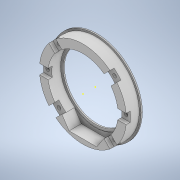
# Autodesk Inventor part: LCDmount
Saved by Autodesk Inventor 2022 (Build 260153000, 153)
## iProperties
Created: 2023-10-26
Part Number: LCDmount
Material: Generisch
Document SubType Name: Modeling
Designer: Marc Panse
Density: 1 g/cm^3
Appearance: Vorgabe
Author: Marc Panse
## iProperties of the stored document LCDmount_3D-Druck.ipt
Created: 2023-10-26
Part Number: LCDmount_3D-Druck
Material: Generisch
Document SubType Name: Modeling
Designer: Marc Panse
Density: 1 g/cm^3
Appearance: Vorgabe
Author: Marc Panse
Autodesk Inventor part; units mm, degrees
ref_plane "YZ Plane" through (0, 0, 0) normal (1, 0, 0) x (0, 1, 0)
ref_plane "XZ Plane" through (0, 0, 0) normal (0, 1, 0) x (-1, 0, 0)
ref_plane "XY Plane" through (0, 0, 0) normal (0, 0, 1) x (1, 0, 0)
sketch "Skizze1" plane through (0, 0, 0) normal (0, 0, 1) x (1, 0, 0)
  circle A0 centre (0, 0) radius 18
  circle A1 centre (0, 0) radius 25
  dimension "d0" = 36
  dimension "d1" = 50
  constraints: 2 centre point, 2 coincident
  measures "d0" diameter of A0
  measures "d1" diameter of A1
extrude "Extrusion1" add sketch "Skizze1" along normal blind 35
sketch "Skizze2" plane through (0, 0, 35) normal (0, 0, 1) x (1, 0, 0)
  circle A0 centre (0, 0) radius 19.3
  line L0 (0, -19.3) -> (0, -21.4)
  line L1 (0, -21.4) -> (-7.65, -21.4)
  line L2 (-7.65, -21.4) -> (7.65, -21.4)
  line L3 (7.65, -21.4) -> (7.65, -17.7191)
  line L4 (-7.65, -21.4) -> (-7.65, -17.7191)
  circle A1 centre (0, 0) radius 25 projected
  circle A2 centre (0, 0) radius 18 projected
  circle A3 centre (0, 0) radius 25 projected
  circle A4 centre (0, 0) radius 18 projected
  circle A5 centre (0, 0) radius 19.3
  dimension "d4" = 38.6
  dimension "d5" = 2.1
  dimension "d6" = 7.65
  dimension "d7" = 90
  dimension "d8" = 15.3
  constraints: 10 end point, 3 point on circle, 2 centre point, 2 coincident, 2 perpendicular, 1 concentric, 1 parallel, 1 point on line, 1 vertical
  measures "d4" diameter of A0
  measures "d5" distance of L0.start L0.end
  measures "d6" distance of L0.end L1.end
  measures "d7" angle of L0 L1
  measures "d8" distance of L1.end L2.end
extrude "Extrusion2" cut sketch "Skizze2" against normal blind 34 contours A0 | A0 L0 L1 L4 | L3 L2 L0 A0 | A2
fillet "Rundung1" radius 4 2 edges at (-7.65, -17.7191, 18) (7.65, -17.7191, 18)
sketch "Skizze3" plane through (0, 0, 35) normal (0, 0, 1) x (1, 0, 0)
  arc A0 (9.65, -16.7143) -> (7.65, -20.1784) centre (11.65, -20.1784) ccw projected
  line L0 (7.65, -20.1784) -> (7.65, -21.4) projected
  line L1 (7.65, -21.4) -> (-7.65, -21.4) projected
  line L2 (-7.65, -21.4) -> (-7.65, -20.1784) projected
  arc A1 (-7.65, -20.1784) -> (-9.65, -16.7143) centre (-11.65, -20.1784) ccw projected
  arc A2 (9.65, -16.7143) -> (-9.65, -16.7143) centre (0, 0) ccw projected
  circle A3 centre (0, 0) radius 25 projected
extrude "Extrusion3" cut sketch "Skizze3" against normal blind 25
sketch "Skizze4" plane through (0, 0, 10) normal (0, 0, 1) x (1, 0, 0)
  circle A0 centre (0, 0) radius 24
  circle A1 centre (0, 0) radius 25 projected
  arc A2 (9.65, -16.7143) -> (7.65, -20.1784) centre (11.65, -20.1784) ccw projected
  line L0 (7.65, -21.4) -> (7.65, -20.1784) projected
  line L1 (-7.65, -21.4) -> (7.65, -21.4) projected
  line L2 (-7.65, -20.1784) -> (-7.65, -21.4) projected
  arc A3 (-7.65, -20.1784) -> (-9.65, -16.7143) centre (-11.65, -20.1784) ccw projected
  arc A4 (9.65, -16.7143) -> (-9.65, -16.7143) centre (0, 0) ccw projected
  dimension "d14" = 48
  constraints: 1 centre point, 1 coincident
  measures "d14" diameter of A0
extrude "Extrusion4" cut sketch "Skizze4" against normal blind 9.25 contours A1
sketch "Skizze5" plane through (0, 0, 10) normal (0, 0, 1) x (1, 0, 0)
  circle A0 centre (0, 0) radius 24 projected
  arc A1 (9.65, -16.7143) -> (7.65, -20.1784) centre (11.65, -20.1784) ccw projected
  line L0 (7.65, -21.4) -> (7.65, -20.1784) projected
  line L1 (-7.65, -21.4) -> (7.65, -21.4) projected
  line L2 (-7.65, -20.1784) -> (-7.65, -21.4) projected
  arc A2 (-7.65, -20.1784) -> (-9.65, -16.7143) centre (-11.65, -20.1784) ccw projected
  arc A3 (9.65, -16.7143) -> (-9.65, -16.7143) centre (0, 0) ccw projected
extrude "Extrusion5" cut sketch "Skizze5" against normal blind 2.2
sketch "Skizze6" plane through (0, 0, 7.8) normal (0, 0, 1) x (1, 0, 0)
  line L0 (30, -2.706) -> (-30, -2.706)
  line L1 (-30, -2.706) -> (-30, 2.706)
  line L2 (-30, 2.706) -> (30, 2.706)
  line L3 (30, 2.706) -> (30, -2.706)
  line L4 (30, -2.706) -> (-30, 2.706) construction
  line L5 (-30, -2.706) -> (30, 2.706) construction
  point P0 (0, 0)
  dimension "d33" = 60
  constraints: 12 end point, 2 midpoint, 2 parallel, 1 horizontal, 1 perpendicular
  measures "d33" distance between parallel lines of L3 L1
extrude "Extrusion6" cut sketch "Skizze6" against normal blind 2.2
sketch "Skizze7" plane through (0, 0, 5.6) normal (0, 0, 1) x (1, 0, 0)
  line L0 (-22.5614, -2.035) -> (-22.5614, 2.035) projected
  line L1 (-22.5614, 0) -> (-19.3, 0)
  arc A0 (-19.1094, 2.706) -> (-19.1094, -2.706) centre (0, 0) ccw projected
  line L2 (-19.3, 0) -> (-24, 0)
  circle A1 centre (0, 0) radius 24 projected
  circle A2 centre (-21.65, 0) radius 0.9
  dimension "d34" = 1.8
  constraints: 4 end point, 2 horizontal, 2 midpoint, 1 centre point, 1 horizontal alignment, 1 point on circle, 1 other
  measures "d34" diameter of A2
extrude "Extrusion7" cut sketch "Skizze7" against normal blind 4 contours A2 L1 | L1 A2
mirror "Spiegeln1" about plane through (0, 0, 0) normal (1, 0, 0) of "Extrusion7"
sketch "Skizze8" plane through (0, 0, 7.8) normal (0, 0, 1) x (1, 0, 0)
  point P0 (0, 0)
pattern_circular "Runde Anordnung1" count 8 over 360 about axis through (0, 0, -10) along (0, 0, 1) of "Extrusion7", "Extrusion6"
sketch "Skizze9" plane through (0, -20.9307, 1.6) normal (0, 0, 1) x (1, 0, 0)
  line L0 (-0.8646, -0.4693) -> (0.8646, -0.4693) projected
  line L1 (-2.706, -0.4693) -> (-0.8646, -0.4693) projected
  line L2 (-2.706, 40.0401) -> (-2.706, 44.7777) projected
  line L3 (2.706, 44.7777) -> (2.706, 40.0401) projected
  arc A0 (2.706, 44.7777) -> (-2.706, 44.7777) centre (0, 20.9307) ccw projected
  arc A1 (2.706, 40.0401) -> (-2.706, 40.0401) centre (0, 20.9307) ccw projected
  arc A2 (-2.706, -2.9163) -> (2.706, -2.9163) centre (0, 20.9307) ccw projected
  line L4 (2.706, -0.4693) -> (2.706, -2.9163) projected
  line L5 (-2.706, -2.9163) -> (-2.706, -0.4693) projected
  line L6 (0.8646, -0.4693) -> (2.706, -0.4693) projected
  arc A3 (-0.8646, -0.4693) -> (0.8646, -0.4693) centre (0, -0.7193) ccw projected
  arc A4 (-0.8646, -0.4693) -> (0.8646, -0.4693) centre (0, -0.7193) ccw projected
extrude "Extrusion8" add sketch "Skizze9" along normal blind 4 contours L0 A3
sketch "Skizze10" plane through (-2.706, -21.4, 5.6) normal (0, 0, 1) x (1, 0, 0)
  line L0 (0, 0) -> (5.412, 0) projected
  line L1 (0, 40.5094) -> (0, 45.247) projected
  line L2 (5.412, 45.247) -> (5.412, 40.5094) projected
  arc A0 (5.412, 45.247) -> (0, 45.247) centre (2.706, 21.4) ccw projected
  arc A1 (5.412, 40.5094) -> (0, 40.5094) centre (2.706, 21.4) ccw projected
  arc A2 (0, -2.447) -> (5.412, -2.447) centre (2.706, 21.4) ccw projected
  line L3 (5.412, 0) -> (5.412, -2.447) projected
  line L4 (0, -2.447) -> (0, 0) projected
extrude "Extrusion9" add sketch "Skizze10" along normal up to surface (2.2 mm away)
sketch "Skizze11" plane through (0, 0, 7.8) normal (0, 0, 1) x (-0.3826834, -0.9238795, 0)
  line L0 (15.7149, 14.7896) -> (16.8435, 15.2571) projected
  arc A0 (11.7491, 15.3117) -> (9.8128, 16.6192) centre (0, 0) ccw projected
  line L1 (16.8435, 15.2571) -> (11.7491, 15.3117)
  line L2 (-18.6903, 4.8128) -> (-23.0673, 6.6258) projected
  arc A1 (9.8128, -16.6192) -> (16.6192, -9.8128) centre (0, 0) ccw projected
  line L3 (9.8128, -16.6192) -> (11.6258, -20.9962) projected
  line L4 (6.6258, -23.0673) -> (4.8128, -18.6903) projected
  arc A2 (-4.8128, -18.6903) -> (4.8128, -18.6903) centre (0, 0) ccw projected
  line L5 (-4.8128, -18.6903) -> (-6.6258, -23.0673) projected
  line L6 (4.8128, 18.6903) -> (6.6258, 23.0673) projected
  line L7 (20.9962, -11.6258) -> (16.6192, -9.8128) projected
  line L8 (18.6903, -4.8128) -> (23.0673, -6.6258) projected
  arc A3 (-9.8128, 16.6192) -> (-16.6192, 9.8128) centre (0, 0) ccw projected
  line L9 (-9.8128, 16.6192) -> (-11.6258, 20.9962) projected
  line L10 (-6.6258, 23.0673) -> (-4.8128, 18.6903) projected
  arc A4 (4.8128, 18.6903) -> (-4.8128, 18.6903) centre (0, 0) ccw projected
  line L11 (-11.6258, -20.9962) -> (-9.8128, -16.6192) projected
  line L12 (11.6258, 20.9962) -> (9.8128, 16.6192) projected
  arc A5 (11.7491, 15.3117) -> (9.8128, 16.6192) centre (0, 0) ccw projected
  arc A6 (11.7491, 15.3117) -> (15.7149, 14.7896) centre (14.1841, 18.4851) ccw projected
  line L13 (16.8435, 15.2571) -> (15.7149, 14.7896) projected
  line L14 (22.6986, 1.1217) -> (16.8435, 15.2571) projected
  line L15 (21.5699, 0.6543) -> (22.6986, 1.1217) projected
  arc A7 (21.5699, 0.6543) -> (19.1349, -2.5192) centre (23.1007, -3.0413) ccw projected
  arc A8 (18.6903, -4.8128) -> (19.1349, -2.5192) centre (0, 0) ccw projected
  line L16 (-20.9962, 11.6258) -> (-16.6192, 9.8128) projected
  arc A9 (-6.6258, -23.0673) -> (6.6258, -23.0673) centre (0, 0) ccw projected
  arc A10 (-18.6903, 4.8128) -> (-9.8128, -16.6192) centre (0, 0) ccw projected
  arc A11 (-23.0673, 6.6258) -> (-11.6258, -20.9962) centre (0, 0) ccw projected
  arc A12 (-11.6258, 20.9962) -> (-20.9962, 11.6258) centre (0, 0) ccw projected
  arc A13 (11.6258, -20.9962) -> (20.9962, -11.6258) centre (0, 0) ccw projected
  arc A14 (6.6258, 23.0673) -> (-6.6258, 23.0673) centre (0, 0) ccw projected
  arc A15 (23.0673, -6.6258) -> (11.6258, 20.9962) centre (0, 0) ccw projected
  point P0 (15.7149, 14.7896)
  constraints: 2 end point
extrude "Extrusion10" cut sketch "Skizze11" against normal up to surface (6.8 mm away) contours A6 L1 L0
mirror "Spiegeln2" about plane through (0, 0, 0) normal (1, 0, 0) of "Extrusion10"
sketch "Skizze12" plane through (0, 0, 7.8) normal (0, 0, 1) x (-0.3826834, -0.9238795, 0)
  point P0 (0, 0)
sketch "Skizze13" plane through (0, 0, 7.8) normal (0, 0, 1) x (1, 0, 0)
  line L0 (-7.65, -21.4) -> (-9.65, -16.7143) projected
  arc A0 (-11.5989, -15.4258) -> (-9.65, -16.7143) centre (0, 0) ccw projected
  line L1 (-11.5989, -15.4258) -> (-14.9489, -18.7758) projected
  arc A1 (-14.9489, -18.7758) -> (14.9489, -18.7758) centre (0, 0) ccw projected
  line L2 (14.9489, -18.7758) -> (11.5989, -15.4258) projected
  arc A2 (9.65, -16.7143) -> (11.5989, -15.4258) centre (0, 0) ccw projected
  line L3 (9.65, -16.7143) -> (7.65, -21.4) projected
  line L4 (-7.65, -21.4) -> (7.65, -21.4) projected
  arc A3 (-11.5989, -15.4258) -> (-9.65, -16.7143) centre (0, 0) ccw projected
  line L5 (7.65, -21.4) -> (-7.65, -21.4) projected
  line L6 (-11.5989, -15.4258) -> (-7.65, -21.4)
  constraints: 2 end point
extrude "Extrusion11" cut sketch "Skizze13" against normal up to surface (6.8 mm away) contours L6 A0 L0
mirror "Spiegeln3" about plane through (0, 0, 0) normal (1, 0, 0) of "Extrusion11"
sketch "Skizze14" plane through (0, 0, 1) normal (0, 0, 1) x (1, 0, 0)
  point P0 (0, 0)
sketch "Skizze15" plane through (0, 0, 7.8) normal (0, 0, 1) x (1, 0, 0)
  circle A0 centre (0, 0) radius 19.375
  dimension "d37" = 38.75
  constraints: 1 centre point, 1 coincident
  measures "d37" diameter of A0
extrude "Extrusion12" cut sketch "Skizze15" against normal up to surface (7.05 mm away)
sketch "Skizze16" plane through (0, 0, 7.8) normal (0, 0, 1) x (1, 0, 0)
  circle A0 centre (-15.3089, 15.3089) radius 0.9 projected
  circle A1 centre (-15.3089, 15.3089) radius 1
  circle A2 centre (-21.65, 0) radius 0.9 projected
  circle A3 centre (-21.65, 0) radius 1
  circle A4 centre (-15.3089, -15.3089) radius 0.9 projected
  circle A5 centre (-15.3089, -15.3089) radius 1
  circle A6 centre (15.3089, -15.3089) radius 0.9 projected
  circle A7 centre (15.3089, -15.3089) radius 1
  circle A8 centre (21.65, 0) radius 0.9 projected
  circle A9 centre (21.65, 0) radius 1
  circle A10 centre (15.3089, 15.3089) radius 0.9 projected
  circle A11 centre (15.3089, 15.3089) radius 1
  point P0 (0, 0)
  dimension "d40" = 2
  dimension "d41" = 2
  dimension "d42" = 2
  dimension "d43" = 2
  dimension "d44" = 2
  dimension "d45" = 2
  constraints: 6 centre point, 6 coincident
  measures "d40" diameter of A1
  measures "d41" diameter of A3
  measures "d42" diameter of A5
  measures "d43" diameter of A7
  measures "d44" diameter of A9
  measures "d45" diameter of A11
extrude "Extrusion13" cut sketch "Skizze16" against normal up to surface (7.05 mm away) contours A0 | A1 | A2 | A3 | A4 | A5 | A7 | A8 | A9 | A11
